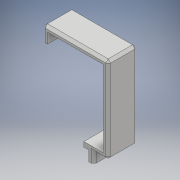
# Autodesk Inventor part: FEMUR2_B
Saved by Autodesk Inventor 2017 (Build 210142000, 142)
## iProperties
Created: 2017-09-24
Part Number: FEMUR2_B
Material: Generic
Document SubType Name: Modeling
Designer: Alexander Miller
Density: 1 g/cm^3
Appearance: Default
Author: Alexander Miller
Autodesk Inventor part; units mm, degrees
ref_plane "YZ Plane" through (0, 0, 0) normal (1, 0, 0) x (0, 1, 0)
ref_plane "XZ Plane" through (0, 0, 0) normal (0, 1, 0) x (-1, 0, 0)
ref_plane "XY Plane" through (0, 0, 0) normal (0, 0, 1) x (1, 0, 0)
sketch "Sketch1" plane through (0, 0, 0) normal (0, 1, 0) x (-1, 0, 0)
  line L0 (21.7482, 13.5362) -> (21.7482, 19.7862)
  line L1 (21.7482, 19.7862) -> (-5.2518, 19.7862)
  line L2 (-5.2518, 19.7862) -> (-5.2518, -15.7138)
  line L3 (-5.2518, -15.7138) -> (0.7482, -15.7138)
  line L4 (0.7482, -15.7138) -> (0.7482, -19.9638)
  line L5 (0.7482, -19.9638) -> (2.7482, -19.9638)
  line L6 (4.7482, -13.7138) -> (-3.2518, -13.7138)
  line L7 (-3.2518, -13.7138) -> (-3.2518, 17.7862)
  line L8 (-3.2518, 17.7862) -> (19.7482, 17.7862)
  line L9 (19.7482, 17.7862) -> (19.7482, 13.5362)
  line L10 (19.7482, 13.5362) -> (21.7482, 13.5362)
  line L11 (4.7482, -13.7138) -> (4.7482, -15.7138)
  line L12 (4.7482, -15.7138) -> (2.7482, -15.7138)
  line L13 (2.7482, -15.7138) -> (2.7482, -19.9638)
  point P0 (0, 0)
  dimension "d1" = 4.25
  dimension "d2" = 2
  dimension "d3" = 2
  dimension "d4" = 2
  dimension "d5" = 2
  dimension "d6" = 2
  dimension "d7" = 23
  dimension "d8" = 2
  dimension "d9" = 4.25
  dimension "d10" = 2
  dimension "d21" = 31.5
  dimension "d22" = 8
  constraints: 28 end point, 11 perpendicular, 2 vertical
  measures "d1" distance of L8.end L9.end
  measures "d2" distance of L9.end L0.start
  measures "d3" distance of L4.end L5.end
  measures "d4" distance between parallel lines of L6 L3
  measures "d5" distance between parallel lines of L8 L1
  measures "d6" distance between parallel lines of L2 L7
  measures "d7" distance of L7.end L8.end
  measures "d8" distance of L11.end L12.end
  measures "d9" distance of L12.end L5.end
  measures "d10" distance of L6.start L11.end
  measures "d21" distance between parallel lines of L8 L6
  measures "d22" distance between parallel lines of L7 L11
extrude "Extrusion1" add sketch "Sketch1" along normal blind 12
sketch "Sketch2" plane through (-21.7482, 0, 13.5362) normal (-1, 0, 0) x (0, 0, 1)
  circle A0 centre (2.5, 6) radius 1
  line L0 (6.25, 0) -> (6.25, 12) projected
  line L1 (0, 0) -> (0, 12) projected
  point P0 (-13.5362, 0)
  point P1 (6.25, 6)
  dimension "d13" = 1.5
  dimension "d14" = 2
  constraints: 1 centre point, 1 horizontal alignment, 1 midpoint
  measures "d13" distance edge to line of A0 L1
  measures "d14" diameter of A0
extrude "Extrusion2" cut sketch "Sketch2" against normal up to surface (2 mm away)
sketch "Sketch3" plane through (-2.7482, 0, -19.9638) normal (-1, 0, 0) x (0, 0, 1)
  circle A0 centre (2.5, 6) radius 1
  line L0 (0, 0) -> (0, 12) projected
  point P0 (19.9638, 0)
  point P1 (0, 6)
  dimension "d17" = 1.5
  dimension "d18" = 2
  constraints: 1 centre point, 1 horizontal alignment, 1 midpoint
  measures "d17" distance edge to line of A0 L0
  measures "d18" diameter of A0
extrude "Extrusion3" cut sketch "Sketch3" against normal up to surface (2 mm away)
chamfer "Chamfer1" distance 1 angle 45 13 edges at (5.2518, 0, 2.0362) (5.2518, 12, 2.0362) (-8.2482, 12, 19.7862) (-8.2482, 0, 19.7862) (-21.7482, 0, 16.6612) (-21.7482, 12, 16.6612) (-21.7482, 6, 19.7862) (5.2518, 6, -15.7138) (2.2518, 12, -15.7138) (2.2518, 0, -15.7138) (-0.7482, 12, -17.8388) (-0.7482, 0, -17.8388) (5.2518, 6, 19.7862)
sketch "Sketch4" plane through (5.2518, 1, -14.7138) normal (1, 0, 0) x (0, 0, -1)
  circle A0 centre (2.75, 5) radius 2.5
  circle A1 centre (2.75, 5) radius 1 projected
  point P0 (-14.7138, -1)
  dimension "d26" = 5
  constraints: 1 centre point, 1 concentric
  measures "d26" diameter of A0
extrude "Extrusion4" cut sketch "Sketch4" against normal up to surface (6 mm away) contours A0 | A1
equation "\"d1\" = -0.5 * servo_A + 0.5 * servo_D"
equation "\"d7\" = servo_E + servo_F"
equation "\"d8\" = servo_F"
equation "\"d9\" = -0.5 * servo_A + 0.5 * servo_D"
equation "\"d21\" = servo_D"
equation "\"d11\" = servo_B"
equation "\"d13\" = servo_L"
equation "\"d14\" = servo_H"
equation "\"d15\" = servo_B"
equation "\"d17\" = servo_L"
equation "\"d18\" = servo_H"
equation "\"d19\" = servo_B"
equation "\"servo_A\" = 23"
equation "\"servo_D\" = 31.5"
equation "\"servo_E\" = 21"
equation "\"servo_F\" = 2"
equation "\"servo_B\" = 12"
equation "\"servo_L\" = 1.5"
equation "\"servo_H\" = 2"
body "Solid1"
